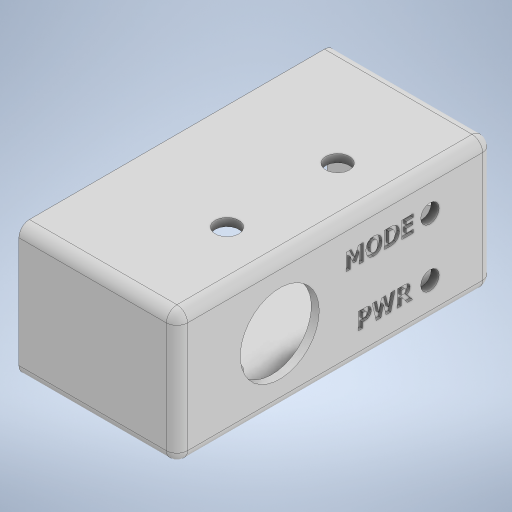
# Autodesk Inventor part: SwitchIO
Saved by Autodesk Inventor 2024.2 (Build 282272000, 272)
## iProperties
Created: 2024-06-01
Part Number: SwitchIO
Material: Generic
Document SubType Name: Modeling
Designer: Robin
Density: 1 g/cm^3
Appearance: Default
Author: Robin
Autodesk Inventor part; units mm, degrees
note: some values were not read from the file. Chosen so that the rebuilt part matches the saved one: direction of "Emboss1".
ref_plane "YZ Plane" through (0, 0, 0) normal (1, 0, 0) x (0, 1, 0)
ref_plane "XZ Plane" through (0, 0, 0) normal (0, 1, 0) x (-1, 0, 0)
ref_plane "XY Plane" through (0, 0, 0) normal (0, 0, 1) x (1, 0, 0)
sketch "Sketch1" plane through (0, 0, 0) normal (0, 1, 0) x (-1, 0, 0)
  line L0 (30, 30) -> (0, 30)
  line L1 (0, 30) -> (0, -30)
  line L2 (0, -30) -> (30, -30)
  line L3 (30, -30) -> (30, 30)
  point P0 (0, 0)
  point P1 (0, 0)
  dimension "d0" = 30
  dimension "d1" = 60
  constraints: 8 end point, 2 parallel, 1 coincident, 1 horizontal, 1 midpoint, 1 perpendicular, 1 vertical alignment
  measures "d0" distance of L1.end L2.end
  measures "d1" distance of L2.end L0.start
extrude "Extrusion1" add sketch "Sketch1" along normal blind 25
shell "Shell2" thickness 1.5 removed faces 1 at (-30, 8.3333, -10)
sketch "Sketch2" plane through (-1.5, 1.5, 28.5) normal (-1, 0, 0) x (0, 0, 1)
  line L0 (0, 22) -> (0, 0) projected
  line L1 (-58.5, -1.5) -> (1.5, -1.5) projected
  circle A0 centre (-18, 11) radius 7.5
  point P0 (0, 11)
  point P1 (-28.5, -1.5)
  dimension "d20" = 15
  dimension "d21" = 18
  constraints: 2 midpoint, 1 centre point, 1 horizontal alignment
  measures "d20" diameter of A0
  measures "d21" distance of point (0, 11) A0.centre
extrude "Extrusion2" cut sketch "Sketch2" against normal blind 25
sketch "Sketch3" plane through (0, 0, 0) normal (0, -1, 0) x (1, 0, 0)
  line L0 (0, 30) -> (0, -30) projected
  point P0 (0, 0)
  point P1 (-10, -10.5)
  point P2 (-10, 10.5)
  point P3 (0, 0)
  point P4 (0, 0)
  dimension "d9" = 21
  dimension "d10" = 10
  dimension "d11" = 10.5
  constraints: 2 midpoint, 1 vertical alignment
  measures "d9" distance of point (-10, 10.5) point (-10, -10.5)
  measures "d10" horizontal distance of point (0, 0) point (-10, -10.5)
  measures "d11" vertical distance of point (0, 0) point (-10, -10.5)
hole "Hole1" at (-10, 0, -10.5) at (-10, 0, 10.5) direction (0, 1, 0) diameter 4.5 end through all both
fillet "Fillet1" radius 2 16 edges at (0, 25, 0) (0, 12.5, -30) (0, 0, 0) (0, 12.5, 30) (-1.5, 23.5, 0) (-1.5, 12.5, 28.5) (-1.5, 1.5, 0) (-1.5, 12.5, -28.5) (-15.75, 23.5, -28.5) (-15.75, 23.5, 28.5) (-15.75, 1.5, 28.5) (-15.75, 1.5, -28.5) (-15, 25, 30) (-15, 0, 30) (-15, 0, -30) (-15, 25, -30)
sketch "Sketch4" plane through (0, 2, -28) normal (1, 0, 0) x (0, 0, -1)
  line L0 (0, 0) -> (-56, 0) projected
  line L1 (-56, 21) -> (0, 21) projected
  line L2 (0, 21) -> (0, 0) projected
  point P0 (-28, -2)
  point P1 (-10, 16)
  point P2 (-10, 5)
  dimension "d22" = 5
  dimension "d23" = 5
  dimension "d24" = 10
  constraints: 1 vertical alignment
  measures "d22" distance from line of L0 point (-10, 5)
  measures "d23" distance from line of L1 point (-10, 16)
  measures "d24" distance from line of L2 point (-10, 16)
hole "Hole2" at (0, 18, -18) at (0, 7, -18) direction (-1, 0, 0) diameter 3.5 end through all
sketch "Sketch5" plane through (-2, 23, -30) normal (0, 0, -1) x (-1, 0, 0)
  line L0 (0, -21) -> (0, 0) projected
  point P0 (-2, -23)
  point P1 (10, -10.5)
  point P2 (0, -10.5)
  point P3 (0, -10.5)
  dimension "d32" = 10
  constraints: 2 midpoint, 1 horizontal alignment
  measures "d32" distance of point (0, -10.5) point (10, -10.5)
hole "Hole3" at (-12, 12.5, -30) direction (0, 0, 1) diameter 8 depth 8 tip angle 118
sketch "Sketch6" plane through (0, 2, -28) normal (1, 0, 0) x (0, 0, -1)
  line L0 (-26.1967, 17.6078) -> (-14.8049, 17.6078) construction
  line L1 (-14.8049, 17.6078) -> (-14.8049, 14.4314) construction
  line L2 (-14.8049, 14.4314) -> (-26.1967, 14.4314) construction
  line L3 (-26.1967, 14.4314) -> (-26.1967, 17.6078) construction
  line L4 (-22.0141, 7.5366) -> (-10.6224, 7.5366) construction
  line L5 (-10.6224, 7.5366) -> (-10.6224, 4.3602) construction
  line L6 (-10.6224, 4.3602) -> (-22.0141, 4.3602) construction
  line L7 (-22.0141, 4.3602) -> (-22.0141, 7.5366) construction
  line L8 (-23.9092, 6.6773) -> (-15.2172, 6.6773) construction
  line L9 (-15.2172, 6.6773) -> (-15.2172, 3.6293) construction
  line L10 (-15.2172, 3.6293) -> (-23.9092, 3.6293) construction
  line L11 (-23.9092, 3.6293) -> (-23.9092, 6.6773) construction
  line L12 (-22.6311, 14.371) -> (-23.4223, 14.371)
  line L13 (-23.4223, 14.371) -> (-23.4223, 16.4723)
  line L14 (-23.4223, 16.4723) -> (-23.9977, 15.116)
  line L15 (-23.9977, 15.116) -> (-24.5423, 15.116)
  line L16 (-24.5423, 15.116) -> (-25.1177, 16.4723)
  line L17 (-25.1177, 16.4723) -> (-25.1177, 14.371)
  line L18 (-25.1177, 14.371) -> (-25.8678, 14.371)
  line L19 (-25.8678, 14.371) -> (-25.8678, 17.541)
  line L20 (-25.8678, 17.541) -> (-24.9508, 17.541)
  line L21 (-24.9508, 17.541) -> (-24.2469, 15.9766)
  line L22 (-24.2469, 15.9766) -> (-23.5481, 17.541)
  line L23 (-23.5481, 17.541) -> (-22.6311, 17.541)
  line L24 (-22.6311, 17.541) -> (-22.6311, 14.371)
  spline S0 degree 2 poles (-19.0886, 15.956) (-19.0886, 15.1853) (-19.9106, 14.3042) (-20.6248, 14.3042) knots 0 0 0 1 2 2 2
  spline S1 degree 2 poles (-20.6248, 14.3042) (-21.3415, 14.3042) (-22.1584, 15.1956) (-22.1584, 15.956) knots 0 0 0 1 2 2 2
  spline S2 degree 2 poles (-22.1584, 15.956) (-22.1584, 16.719) (-21.3415, 17.6078) (-20.6248, 17.6078) knots 0 0 0 1 2 2 2
  spline S3 degree 2 poles (-20.6248, 17.6078) (-19.9106, 17.6078) (-19.0886, 16.7241) (-19.0886, 15.956) knots 0 0 0 1 2 2 2
  spline S4 degree 2 poles (-19.9106, 15.956) (-19.9106, 16.2411) (-20.0262, 16.6393) (-20.1264, 16.7652) knots 0 0 0 1 2 2 2
  spline S5 degree 2 poles (-20.1264, 16.7652) (-20.2266, 16.8962) (-20.4835, 17.0092) (-20.6222, 17.0092) knots 0 0 0 1 2 2 2
  spline S6 degree 2 poles (-20.6222, 17.0092) (-20.7686, 17.0092) (-21.0075, 16.9039) (-21.118, 16.7703) knots 0 0 0 1 2 2 2
  spline S7 degree 2 poles (-21.118, 16.7703) (-21.2156, 16.647) (-21.3363, 16.2386) (-21.3363, 15.956) knots 0 0 0 1 2 2 2
  spline S8 degree 2 poles (-21.3363, 15.956) (-21.3363, 15.6631) (-21.2207, 15.2778) (-21.1206, 15.1468) knots 0 0 0 1 2 2 2
  spline S9 degree 2 poles (-21.1206, 15.1468) (-21.0204, 15.0158) (-20.7609, 14.9028) (-20.6222, 14.9028) knots 0 0 0 1 2 2 2
  spline S10 degree 2 poles (-20.6222, 14.9028) (-20.4809, 14.9028) (-20.2189, 15.0235) (-20.1238, 15.1519) knots 0 0 0 1 2 2 2
  spline S11 degree 2 poles (-20.1238, 15.1519) (-20.0211, 15.2907) (-19.9106, 15.658) (-19.9106, 15.956) knots 0 0 0 1 2 2 2
  spline S12 degree 2 poles (-15.7876, 15.9534) (-15.7876, 15.509) (-16.1755, 14.8103) (-16.4709, 14.6228) knots 0 0 0 1 2 2 2
  spline S13 degree 2 poles (-16.4709, 14.6228) (-16.7175, 14.4635) (-17.2981, 14.371) (-17.6243, 14.371) knots 0 0 0 1 2 2 2
  line L25 (-17.6243, 14.371) -> (-18.6159, 14.371)
  line L26 (-18.6159, 14.371) -> (-18.6159, 17.541)
  line L27 (-18.6159, 17.541) -> (-17.6346, 17.541)
  spline S14 degree 2 poles (-17.6346, 17.541) (-17.3006, 17.541) (-16.7175, 17.4562) (-16.4606, 17.2918) knots 0 0 0 1 2 2 2
  spline S15 degree 2 poles (-16.4606, 17.2918) (-16.1498, 17.0914) (-15.7876, 16.4133) (-15.7876, 15.9534) knots 0 0 0 1 2 2 2
  spline S16 degree 2 poles (-16.6045, 15.9586) (-16.6045, 16.272) (-16.8202, 16.719) (-17.0412, 16.8448) knots 0 0 0 1 2 2 2
  spline S17 degree 2 poles (-17.0412, 16.8448) (-17.203, 16.9322) (-17.5575, 16.9502) (-17.8041, 16.9502) knots 0 0 0 1 2 2 2
  line L28 (-17.8041, 16.9502) -> (-17.8195, 16.9502)
  line L29 (-17.8195, 16.9502) -> (-17.8195, 14.9644)
  line L30 (-17.8195, 14.9644) -> (-17.8041, 14.9644)
  spline S18 degree 2 poles (-17.8041, 14.9644) (-17.537, 14.9644) (-17.1696, 14.9824) (-17.0026, 15.0877) knots 0 0 0 1 2 2 2
  spline S19 degree 2 poles (-17.0026, 15.0877) (-16.8074, 15.211) (-16.6045, 15.6452) (-16.6045, 15.9586) knots 0 0 0 1 2 2 2
  line L31 (-15.3149, 14.371) -> (-15.3149, 17.541)
  line L32 (-15.3149, 17.541) -> (-13.1724, 17.541)
  line L33 (-13.1724, 17.541) -> (-13.1724, 16.9373)
  line L34 (-13.1724, 16.9373) -> (-14.5237, 16.9373)
  line L35 (-14.5237, 16.9373) -> (-14.5237, 16.3799)
  line L36 (-14.5237, 16.3799) -> (-13.2778, 16.3799)
  line L37 (-13.2778, 16.3799) -> (-13.2778, 15.7762)
  line L38 (-13.2778, 15.7762) -> (-14.5237, 15.7762)
  line L39 (-14.5237, 15.7762) -> (-14.5237, 14.9747)
  line L40 (-14.5237, 14.9747) -> (-13.1724, 14.9747)
  line L41 (-13.1724, 14.9747) -> (-13.1724, 14.371)
  line L42 (-13.1724, 14.371) -> (-15.3149, 14.371)
  spline S20 degree 2 poles (-21.1425, 5.678) (-21.1425, 5.4571) (-21.2838, 5.0563) (-21.4148, 4.9227) knots 0 0 0 1 2 2 2
  spline S21 degree 2 poles (-21.4148, 4.9227) (-21.4944, 4.838) (-21.6897, 4.6992) (-21.8053, 4.6504) knots 0 0 0 1 2 2 2
  spline S22 degree 2 poles (-21.8053, 4.6504) (-21.9234, 4.6016) (-22.1983, 4.5451) (-22.3678, 4.5451) knots 0 0 0 1 2 2 2
  line L43 (-22.3678, 4.5451) -> (-22.784, 4.5451)
  line L44 (-22.784, 4.5451) -> (-22.784, 3.5073)
  line L45 (-22.784, 3.5073) -> (-23.5804, 3.5073)
  line L46 (-23.5804, 3.5073) -> (-23.5804, 6.6773)
  line L47 (-23.5804, 6.6773) -> (-22.3499, 6.6773)
  spline S23 degree 2 poles (-22.3499, 6.6773) (-22.0776, 6.6773) (-21.6794, 6.5771) (-21.5175, 6.4692) knots 0 0 0 1 2 2 2
  spline S24 degree 2 poles (-21.5175, 6.4692) (-21.3377, 6.3485) (-21.1425, 5.9529) (-21.1425, 5.678) knots 0 0 0 1 2 2 2
  spline S25 degree 2 poles (-21.9594, 5.6574) (-21.9594, 5.7936) (-22.0878, 5.9862) (-22.1752, 6.0222) knots 0 0 0 1 2 2 2
  spline S26 degree 2 poles (-22.1752, 6.0222) (-22.2882, 6.071) (-22.4937, 6.0864) (-22.671, 6.0864) knots 0 0 0 1 2 2 2
  line L48 (-22.671, 6.0864) -> (-22.784, 6.0864)
  line L49 (-22.784, 6.0864) -> (-22.784, 5.1359)
  line L50 (-22.784, 5.1359) -> (-22.7275, 5.1359)
  spline S27 degree 2 poles (-22.7275, 5.1359) (-22.617, 5.1359) (-22.4167, 5.1411) (-22.3422, 5.1539) knots 0 0 0 1 2 2 2
  spline S28 degree 2 poles (-22.3422, 5.1539) (-22.2779, 5.1642) (-22.1366, 5.2259) (-22.0981, 5.2644) knots 0 0 0 1 2 2 2
  spline S29 degree 2 poles (-22.0981, 5.2644) (-22.0159, 5.3415) (-21.9594, 5.5136) (-21.9594, 5.6574) knots 0 0 0 1 2 2 2
  line L51 (-16.629, 6.6773) -> (-17.4305, 3.5073)
  line L52 (-17.4305, 3.5073) -> (-18.3039, 3.5073)
  line L53 (-18.3039, 3.5073) -> (-18.8125, 5.4673)
  line L54 (-18.8125, 5.4673) -> (-19.3032, 3.5073)
  line L55 (-19.3032, 3.5073) -> (-20.1792, 3.5073)
  line L56 (-20.1792, 3.5073) -> (-20.9807, 6.6773)
  line L57 (-20.9807, 6.6773) -> (-20.1535, 6.6773)
  line L58 (-20.1535, 6.6773) -> (-19.7168, 4.5554)
  line L59 (-19.7168, 4.5554) -> (-19.1876, 6.6773)
  line L60 (-19.1876, 6.6773) -> (-18.3964, 6.6773)
  line L61 (-18.3964, 6.6773) -> (-17.8929, 4.5528)
  line L62 (-17.8929, 4.5528) -> (-17.4356, 6.6773)
  line L63 (-17.4356, 6.6773) -> (-16.629, 6.6773)
  line L64 (-13.3074, 3.5073) -> (-14.2759, 3.5073)
  line L65 (-14.2759, 3.5073) -> (-15.157, 4.671)
  line L66 (-15.157, 4.671) -> (-15.4447, 4.671)
  line L67 (-15.4447, 4.671) -> (-15.4447, 3.5073)
  line L68 (-15.4447, 3.5073) -> (-16.2359, 3.5073)
  line L69 (-16.2359, 3.5073) -> (-16.2359, 6.6773)
  line L70 (-16.2359, 6.6773) -> (-14.9618, 6.6773)
  spline S30 degree 2 poles (-14.9618, 6.6773) (-14.6972, 6.6773) (-14.3067, 6.6105) (-14.1397, 6.5077) knots 0 0 0 1 2 2 2
  spline S31 degree 2 poles (-14.1397, 6.5077) (-13.9702, 6.3998) (-13.7698, 6.0633) (-13.7698, 5.8064) knots 0 0 0 1 2 2 2
  spline S32 degree 2 poles (-13.7698, 5.8064) (-13.7698, 5.4442) (-14.0986, 4.9895) (-14.3735, 4.8559) knots 0 0 0 1 2 2 2
  line L71 (-14.3735, 4.8559) -> (-13.3074, 3.5073)
  spline S33 degree 2 poles (-14.5867, 5.7062) (-14.5867, 5.827) (-14.6792, 5.9991) (-14.7845, 6.0453) knots 0 0 0 1 2 2 2
  spline S34 degree 2 poles (-14.7845, 6.0453) (-14.859, 6.0762) (-15.0414, 6.0941) (-15.1775, 6.0941) knots 0 0 0 1 2 2 2
  line L72 (-15.1775, 6.0941) -> (-15.4447, 6.0941)
  line L73 (-15.4447, 6.0941) -> (-15.4447, 5.2413)
  line L74 (-15.4447, 5.2413) -> (-15.2161, 5.2413)
  spline S35 degree 2 poles (-15.2161, 5.2413) (-15.0517, 5.2413) (-14.8179, 5.2824) (-14.7383, 5.3466) knots 0 0 0 1 2 2 2
  spline S36 degree 2 poles (-14.7383, 5.3466) (-14.6612, 5.4083) (-14.5867, 5.5727) (-14.5867, 5.7062) knots 0 0 0 1 2 2 2
  point P0 (-28, -2)
  constraints: 5 other
emboss "Emboss1" sketch "Sketch6" operation cut depth 0.5 direction (-1, 0, 0)
body "Solid1"
